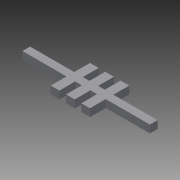
# Autodesk Inventor part: link1
Saved by Autodesk Inventor 2014 SP1 (Build 180222100, 222)
## iProperties
Created: 2015-02-17
Part Number: link1
Material: Generic
Document SubType Name: Modeling
Designer: Erin
Density: 1 g/cm^3
Appearance: Default
Author: Erin
Autodesk Inventor part; units mm, degrees
ref_plane "YZ Plane" through (0, 0, 0) normal (1, 0, 0) x (0, 1, 0)
ref_plane "XZ Plane" through (0, 0, 0) normal (0, 1, 0) x (-1, 0, 0)
ref_plane "XY Plane" through (0, 0, 0) normal (0, 0, 1) x (1, 0, 0)
sketch "tabs" plane through (0, 0, 0) normal (0, 0, 1) x (1, 0, 0)
  line L0 (15.6175, 17.0118) -> (18.7675, 17.0118)
  line L1 (18.7675, 17.0118) -> (18.7675, 10.7868)
  line L2 (18.7675, 10.7868) -> (15.6175, 10.7868)
  line L3 (15.6175, 10.7868) -> (15.6175, 17.0118)
  line L4 (21.8175, 17.0118) -> (24.9675, 17.0118)
  line L5 (24.9675, 17.0118) -> (24.9675, 10.7868)
  line L6 (24.9675, 10.7868) -> (21.8175, 10.7868)
  line L7 (21.8175, 10.7868) -> (21.8175, 17.0118)
  line L8 (28.0175, 17.0118) -> (31.1675, 17.0118)
  line L9 (31.1675, 17.0118) -> (31.1675, 10.7868)
  line L10 (31.1675, 10.7868) -> (28.0175, 10.7868)
  line L11 (28.0175, 10.7868) -> (28.0175, 17.0118)
  line L12 (23.3925, 10.7868) -> (23.3925, 8.8536) construction
  point P0 (23.3925, 12.1901)
  dimension "d2" = 3.15
  dimension "d3" = 3.05
  dimension "d4" = 3.05
  dimension "d5" = 6.225
  measures "d2" distance of L1.end L2.end
  measures "d3" distance between parallel lines of L7 L1
  measures "d4" distance between parallel lines of L11 L5
  measures "d5" distance of L2.end L0.start
sketch "Sketch1" plane through (0, 0, 0) normal (0, 0, 1) x (1, 0, 0)
  line L0 (-25, 1.55) -> (25, 1.55)
  line L1 (25, 1.55) -> (25, -1.55)
  line L2 (25, -1.55) -> (-25, -1.55)
  line L3 (-25, -1.55) -> (-25, 1.55)
  line L4 (0, 16.9043) -> (0, -20.0235) construction
  line L5 (-32.3473, 0) -> (40.4078, 0) construction
  line L6 (-7.775, 7.775) -> (-4.625, 7.775)
  line L7 (-4.625, 7.775) -> (-4.625, 1.55)
  line L8 (-4.625, 1.55) -> (-7.775, 1.55)
  line L9 (-7.775, 1.55) -> (-7.775, 7.775)
  line L10 (-1.575, 7.775) -> (1.575, 7.775)
  line L11 (1.575, 7.775) -> (1.575, 1.55)
  line L12 (1.575, 1.55) -> (-1.575, 1.55)
  line L13 (-1.575, 1.55) -> (-1.575, 7.775)
  line L14 (4.625, 7.775) -> (7.775, 7.775)
  line L15 (7.775, 7.775) -> (7.775, 1.55)
  line L16 (7.775, 1.55) -> (4.625, 1.55)
  line L17 (4.625, 1.55) -> (4.625, 7.775)
  line L18 (0, 1.55) -> (0, -0.3832) construction
  line L19 (-7.775, -1.55) -> (-4.625, -1.55)
  line L20 (-4.625, -1.55) -> (-4.625, -7.775)
  line L21 (-4.625, -7.775) -> (-7.775, -7.775)
  line L22 (-7.775, -7.775) -> (-7.775, -1.55)
  line L23 (-1.575, -1.55) -> (1.575, -1.55)
  line L24 (1.575, -1.55) -> (1.575, -7.775)
  line L25 (1.575, -7.775) -> (-1.575, -7.775)
  line L26 (-1.575, -7.775) -> (-1.575, -1.55)
  line L27 (4.625, -1.55) -> (7.775, -1.55)
  line L28 (7.775, -1.55) -> (7.775, -7.775)
  line L29 (7.775, -7.775) -> (4.625, -7.775)
  line L30 (4.625, -7.775) -> (4.625, -1.55)
  line L31 (0, -7.775) -> (0, -9.7082) construction
  point P0 (0, 0)
  point P1 (25, 0)
  dimension "d0" = 50
  dimension "d1" = 3.1
  constraints: 12 end point, 4 horizontal, 3 parallel, 3 vertical, 2 midpoint, 2 perpendicular, 1 horizontal alignment, 1 vertical alignment
  measures "d0" distance of L1.end L2.end
  measures "d1" distance of L0.end L1.end
extrude "Extrusion1" add sketch "Sketch1" along normal blind 3.1
equation "\"d2\" = mat + kerf"
equation "\"d3\" = mat - kerf"
equation "\"d4\" = mat - kerf"
equation "\"d5\" = 2 * mat + 0.5 * kerf"
equation "\"d1\" = mat"
equation "\"d6\" = mat"
equation "\"mat\" = 3.1"
equation "\"kerf\" = 0.05"
body "Solid1"
